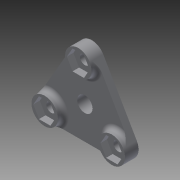
# Autodesk Inventor part: triangle_2
Saved by Autodesk Inventor 2013 (Build 170138000, 138)
## iProperties
Created: 2013-02-11
Part Number: triangle_2
Material: Generic
Document SubType Name: Modeling
Designer: Brad
Density: 1 g/cm^3
Author: Brad
Autodesk Inventor part; units mm, degrees
ref_plane "YZ Plane" through (0, 0, 0) normal (1, 0, 0) x (0, 1, 0)
ref_plane "XZ Plane" through (0, 0, 0) normal (0, 1, 0) x (-1, 0, 0)
ref_plane "XY Plane" through (0, 0, 0) normal (0, 0, 1) x (1, 0, 0)
sketch "Sketch1" plane through (0, 0, 0) normal (0, 0, 1) x (1, 0, 0)
  line L0 (0, 17.609183) -> (15.25, -8.804592)
  line L1 (15.25, -8.804592) -> (-15.25, -8.804592)
  line L2 (-15.25, -8.804592) -> (0, 17.609183)
  circle A0 centre (-15.25, -8.804592) radius 2.25
  circle A1 centre (15.25, -8.804592) radius 2.25
  circle A2 centre (0, 17.609183) radius 2.25
  circle A3 centre (0, 0) radius 3.5
  circle A4 centre (-15.25, -8.804592) radius 6
  circle A5 centre (15.25, -8.804592) radius 6
  circle A6 centre (0, 17.609183) radius 6
  line L3 (5.196152, 20.609183) -> (20.446152, -5.804592)
  line L4 (15.25, -14.804592) -> (-15.25, -14.804592)
  line L5 (-20.446152, -5.804592) -> (-5.196152, 20.609183)
  dimension "d7" = 30.5
  dimension "d8" = 4.5
  dimension "d11" = 360
  dimension "d13" = 7
  dimension "d14" = 12
  dimension "d17" = 360
  dimension "d19" = 6
  constraints: 12 end point, 7 centre point, 6 point on circle, 4 coincident, 21 other
  measures "d7" distance of L0.start L0.end
  measures "d8" diameter of A0
  measures "d13" diameter of A3
  measures "d14" diameter of A4
  measures "d19" distance between parallel lines of L2 L5
extrude "Extrusion1" add sketch "Sketch1" along normal blind 3.175 contours A2 L2 A6 L0 | L0 A6 L2 A2 | A6 L3 A5 L0 | L0 A5 L1 A4 L2 A6 | L2 A4 L5 A6 | A5 L1 A1 L0 | L0 A1 L1 A5 | A4 L1 A0 L2 | L2 A0 L1 A4 | A5 L4 A4 L1
sketch "Sketch2" plane through (0, 0, 0) normal (0, 0, -1) x (-1, 0, 0)
  circle A0 centre (0, 0) radius 3.5 projected
  circle A1 centre (0, 0) radius 6.5
  circle A2 centre (0, 0) radius 3.5
  dimension "d22" = 13
  constraints: 2 centre point, 2 coincident, 1 concentric
  measures "d22" diameter of A1
extrude "Extrusion2" add sketch "Sketch2" along normal blind 4.5
fillet "Fillet1" radius 3 1 edges at (6.5, 0, 0)
sketch "Sketch4" plane through (0, 0, 3.175) normal (0, 0, 1) x (1, 0, 0)
  arc A0 (5.196152, 20.609183) -> (-5.196152, 20.609183) centre (0, 17.609183) ccw
  line L0 (5.196152, 17.609183) -> (2.598076, 13.109183)
  line L1 (2.598076, 13.109183) -> (-2.598076, 13.109183)
  line L2 (-2.598076, 13.109183) -> (-5.196152, 17.609183)
  line L3 (-5.196152, 17.609183) -> (-2.598076, 22.109183)
  line L4 (-2.598076, 22.109183) -> (2.598076, 22.109183)
  line L5 (2.598076, 22.109183) -> (5.196152, 17.609183)
  circle A1 centre (0, 17.609183) radius 6
  line L6 (20.446152, -8.804592) -> (17.848076, -13.304592)
  line L7 (17.848076, -13.304592) -> (12.651924, -13.304592)
  line L8 (12.651924, -13.304592) -> (10.053848, -8.804592)
  line L9 (10.053848, -8.804592) -> (12.651924, -4.304592)
  line L10 (12.651924, -4.304592) -> (17.848076, -4.304592)
  line L11 (17.848076, -4.304592) -> (20.446152, -8.804592)
  circle A2 centre (15.25, -8.804592) radius 6
  line L12 (-10.053848, -8.804592) -> (-12.651924, -13.304592)
  line L13 (-12.651924, -13.304592) -> (-17.848076, -13.304592)
  line L14 (-17.848076, -13.304592) -> (-20.446152, -8.804592)
  line L15 (-20.446152, -8.804592) -> (-17.848076, -4.304592)
  line L16 (-17.848076, -4.304592) -> (-12.651924, -4.304592)
  line L17 (-12.651924, -4.304592) -> (-10.053848, -8.804592)
  circle A3 centre (-15.25, -8.804592) radius 6
  dimension "d31" = 9
  dimension "d32" = 9
  dimension "d33" = 9
  constraints: 36 end point, 3 centre point, 2 coincident, 1 concentric, 13 other
  measures "d31" distance between parallel lines of L1 L4
  measures "d32" distance between parallel lines of L7 L10
  measures "d33" distance between parallel lines of L13 L16
extrude "Extrusion4" add sketch "Sketch4" along normal blind 3
fillet "Fillet3" radius 2 5 edges at (-11.0074, -13.0472, 3.175) (-13.6971, -3.009, 3.175) (5.7956, 19.1621, 3.175) (-1.5529, 11.8136, 3.175) (10.0538, -5.8046, 3.175)
body "Solid1"
